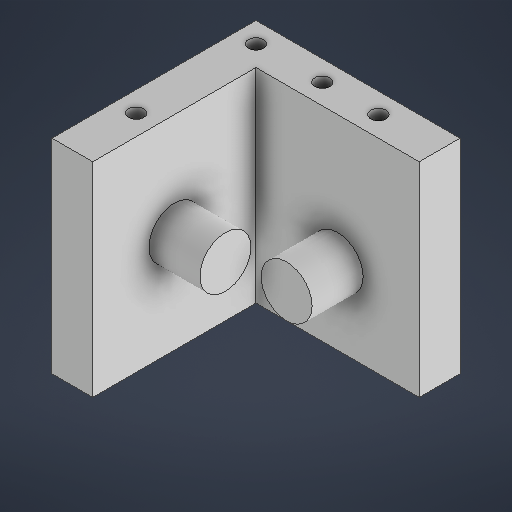
# Autodesk Inventor part: Non-ThorLabs Galvo
Saved by Autodesk Inventor 2025 (Build 290162000, 162)
## iProperties
Created: 2024-06-10
Part Number: Non-ThorLabs Galvo
Material: Generic
Document SubType Name: Modeling
Designer: mayhe
Density: 1 g/cm^3
Appearance: Default
Author: mayhe
Autodesk Inventor part; units mm, degrees
ref_plane "YZ Plane" through (0, 0, 0) normal (1, 0, 0) x (0, 1, 0)
ref_plane "XZ Plane" through (0, 0, 0) normal (0, 1, 0) x (-1, 0, 0)
ref_plane "XY Plane" through (0, 0, 0) normal (0, 0, 1) x (1, 0, 0)
sketch "Sketch1" plane through (0, 0, 0) normal (0, 1, 0) x (-1, 0, 0)
  line L0 (-20, 4) -> (20, 4)
  line L1 (20, 4) -> (20, -4)
  line L2 (20, -4) -> (-20, -4)
  line L3 (-20, -4) -> (-20, 4)
  line L4 (-20, 4) -> (20, -4) construction
  line L5 (20, 4) -> (-20, -4) construction
  line L6 (20, -4) -> (12, -4)
  line L7 (12, -4) -> (12, 36)
  line L8 (12, 36) -> (20, 36)
  line L9 (20, 36) -> (20, -4)
  point P0 (0, 0)
  point P1 (12, 4)
  dimension "d0" = 40
  dimension "d1" = 8
  dimension "d2" = 8
  dimension "d3" = 40
  constraints: 20 end point, 4 parallel, 2 horizontal, 2 midpoint, 2 perpendicular
  measures "d0" distance of L1.end L2.end
  measures "d1" distance of L0.end L1.end
  measures "d2" distance of L7.end L8.end
  measures "d3" distance of L6.end L7.end
extrude "Extrusion1" add sketch "Sketch1" along normal blind 40
sketch "Sketch2" plane through (0, 40, 0) normal (0, 1, 0) x (1, 0, 0)
  circle A0 centre (8, 0) radius 2.5
  circle A1 centre (-3, 0) radius 2.5
  circle A2 centre (-16, 0) radius 2.5
  circle A3 centre (-16, -23.5) radius 2.5
  line L0 (20, -4) -> (20, 4) projected
  line L1 (-20, -36) -> (-12, -36) projected
  point P0 (0, 0)
  point P1 (-16, -36)
  point P2 (-16, -36)
  point P3 (20, 0)
  point P4 (-16, -36)
  point P5 (20, 0)
  dimension "d6" = 5
  dimension "d7" = 5
  dimension "d8" = 5
  dimension "d9" = 5
  dimension "d10" = 12
  dimension "d21" = 12.5
  dimension "d22" = 23
  constraints: 5 midpoint, 4 centre point, 3 horizontal alignment, 3 vertical alignment
  measures "d6" diameter of A0
  measures "d7" diameter of A1
  measures "d8" diameter of A2
  measures "d9" diameter of A3
  measures "d10" distance from line of L0 A0.centre
  measures "d21" distance from line of L1 A3.centre
  measures "d22" distance from line of A1.centre L0
hole "Hole1" at (-16, 40, 23.5) at (-16, 40, 0) at (-3, 40, 0) at (8, 40, 0) direction (0, -1, 0) diameter 3 depth 11 tip angle 118
sketch "Sketch3" plane through (-12, 0, 36) normal (1, 0, 0) x (0, 0, -1)
  circle A0 centre (16, 20) radius 5
  line L0 (0, 0) -> (0, 40) projected
  point P0 (36, 0)
  dimension "d23" = 10
  dimension "d31" = 16
  constraints: 1 centre point
  measures "d23" diameter of A0
  measures "d31" distance from line of L0 A0.centre
extrude "Extrusion2" add sketch "Sketch3" along normal blind 10
sketch "Sketch4" plane through (-12, 0, 4) normal (0, 0, 1) x (1, 0, 0)
  circle A0 centre (16, 15) radius 5
  line L0 (0, 0) -> (32, 0) projected
  line L1 (32, 0) -> (32, 40) projected
  point P0 (12, 0)
  dimension "d26" = 10
  dimension "d27" = 15
  dimension "d28" = 16
  constraints: 1 centre point
  measures "d26" diameter of A0
  measures "d27" distance from line of L0 A0.centre
  measures "d28" distance from line of L1 A0.centre
extrude "Extrusion3" add sketch "Sketch4" along normal blind 10
equation "\"d19\" = d11"
equation "\"d11\" = 11"
body "Solid1"
